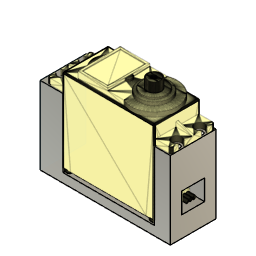
MG996R bracket(bairing) v1 (Autodesk Fusion 360 design; units mm, degrees)
Autodesk Fusion 360 part; units mm, degrees
other "基準メッシュ フィーチャ1"
other "修正1"
other "修正2"
sketch "スケッチ1" plane through (0, 0, 0) normal (0, 0, 1) x (1, 0, 0)
other "修正3"
sketch "スケッチ2" plane through (0, 0, 0) normal (0, 0, 1) x (1, 0, 0)
  line L0 (-20, 10) -> (20, 10)
  line L1 (20, 10) -> (20, -10)
  line L2 (20, -10) -> (-20, -10)
  line L3 (-20, -10) -> (-20, 10)
  line L4 (-20, 10) -> (20, -10) construction
  line L5 (20, 10) -> (-20, -10) construction
  line L6 (20, -10) -> (27, -10)
  line L7 (27, -10) -> (27, 10)
  line L8 (27, 10) -> (20, 10)
  line L9 (20, 10) -> (20, -10)
  line L10 (-20, -10) -> (-27, -10)
  line L11 (-27, -10) -> (-27, 10)
  line L12 (-27, 10) -> (-20, 10)
  line L13 (-20, 10) -> (-20, -10)
  dimension "d1" = 7
  dimension "d2" = 20
  dimension "d3" = 7
  dimension "d4" = 20
  constraint horizontal L0
  constraint perpendicular L0 L1
  constraint parallel L0 L2
  constraint parallel L1 L3
  constraint coincident L4 origin
  constraint coincident L5 origin
  constraint horizontal L6
  constraint vertical L7
  constraint horizontal L8
  constraint vertical L9
  constraint horizontal L10
  constraint vertical L11
  constraint horizontal L12
  constraint vertical L13
  measures "d1" distance of L1.end L6.end
  measures "d2" distance of L1.end L0.end
  measures "d3" distance of L2.end L10.end
  measures "d4" distance of L2.end L0.start
extrude "押し出し1" add sketch "スケッチ2" along normal blind 3
sketch "スケッチ3" plane through (0, 0, 3) normal (0, 0, 1) x (-1, 0, 0)
  line L0 (27, 10) -> (-27, 10)
  line L1 (-27, 10) -> (-27, -10)
  line L2 (-27, -10) -> (27, -10)
  line L3 (27, -10) -> (27, 10)
  line L4 (27, 10) -> (20, 10)
  line L5 (20, 10) -> (20, -10)
  line L6 (20, -10) -> (27, -10)
  line L7 (27, -10) -> (27, 10)
  line L8 (-27, 10) -> (-20, 10)
  line L9 (-20, 10) -> (-20, -10)
  line L10 (-20, -10) -> (-27, -10)
  line L11 (-27, -10) -> (-27, 10)
  constraint horizontal L4
  constraint vertical L5
  constraint horizontal L6
  constraint vertical L7
  constraint coincident L2 L5.end
  constraint coincident L0.start L3.end
  constraint horizontal L8
  constraint vertical L9
  constraint horizontal L10
  constraint vertical L11
  constraint coincident L0.end L1.start
extrude "押し出し2" add sketch "スケッチ3" along normal blind 5 contours L0 L2 L3 L4 L5 L6 L7 | L0 L1 L2 L8 L9 L10 L11
sketch "スケッチ4" plane through (0, 0, 8) normal (0, 0, 1) x (-1, 0, 0)
  line L0 (-27, -10) -> (-20, -10)
  line L1 (-20, -10) -> (-20, 10)
  line L2 (-20, 10) -> (-27, 10)
  line L3 (-27, 10) -> (-27, -10)
  line L4 (-20, 10) -> (-27, 10)
  line L5 (-27, 10) -> (-27, 5)
  line L6 (-27, 5) -> (-20, 5)
  line L7 (-20, 5) -> (-20, 10)
  line L8 (-27, -10) -> (-20, -10)
  line L9 (-20, -10) -> (-20, -5)
  line L10 (-20, -5) -> (-27, -5)
  line L11 (-27, -5) -> (-27, -10)
  dimension "d9" = 7
  dimension "d10" = 5
  constraint horizontal L4
  constraint vertical L5
  constraint horizontal L6
  constraint vertical L7
  constraint coincident L3 L5.end
  constraint coincident L1.end L2.start
  constraint horizontal L8
  constraint vertical L9
  constraint horizontal L10
  constraint vertical L11
  constraint coincident L0.start L3.end
  measures "d9" distance of L0.start L0.end
  measures "d10" distance of L0.start L10.end
extrude "押し出し3" add sketch "スケッチ4" along normal blind 9 contours L0 L1 L3 L8 L9 L10 L11 | L1 L2 L3 L4 L5 L6 L7
sketch "スケッチ5" plane through (0, 0, 17) normal (0, 0, 1) x (-1, 0, 0)
  line L0 (-27, -5) -> (-27, -10)
  line L1 (-27, -10) -> (-20, -10)
  line L2 (-20, -10) -> (-20, -5)
  line L3 (-20, -5) -> (-27, -5)
  line L4 (-20, 10) -> (-27, 10)
  line L5 (-27, 10) -> (-27, -10)
  line L6 (-27, -10) -> (-20, -10)
  line L7 (-20, -10) -> (-20, 10)
  constraint horizontal L4
  constraint vertical L5
  constraint horizontal L6
  constraint vertical L7
  constraint coincident L0.end L1.start
extrude "押し出し4" add sketch "スケッチ5" along normal blind 16
extrude "押し出し5" add 1 faces at (-22.3333, 3.3333, 8) along direction (0, 0, 1) blind 25
sketch "スケッチ6" plane through (0, 0, 33) normal (0, 0, 1) x (-1, 0, 0)
  line L0 (-20, -10) -> (-20, 10)
  line L1 (-20, 10) -> (-27, 10)
  line L2 (-27, 10) -> (-27, -10)
  line L3 (-27, -10) -> (-20, -10)
  circle A0 centre (-25, 5) radius 1.5
  circle A1 centre (-25, -5) radius 1.5
  circle A2 centre (24.95, 5.2) radius 1.5
  circle A3 centre (25, -4.8) radius 1.5
  dimension "d17" = 3
  dimension "d18" = 3
  dimension "d19" = 3
  dimension "d20" = 3
  measures "d17" diameter of A0
  measures "d18" diameter of A1
  measures "d19" diameter of A2
  measures "d20" diameter of A3
extrude "押し出し6" cut sketch "スケッチ6" against normal blind 5 contours A0 | A1 | A2 | A3
thread "ねじ1" "ISO Metric profile 3.0 M3x0.5 M3x0.5 6H" major diameter 3.086 minor diameter 2.529 pitch 0.5 angle 60 resizes the face on face at (-26.4981, 4.8748, 29.6667)
thread "ねじ2" "ISO Metric profile 3.0 M3x0.5 M3x0.5 6H" major diameter 3.086 minor diameter 2.529 pitch 0.5 angle 60 resizes the face on face at (-26.4481, -5.1252, 29.6667)
thread "ねじ3" "ISO Metric profile 3.0 M3x0.5 M3x0.5 6H" major diameter 3.086 minor diameter 2.529 pitch 0.5 angle 60 resizes the face on face at (23.5019, -4.9252, 29.6667) on face at (23.5019, 5.0748, 29.6667)
extrude "押し出し7" add 1 faces at (-9, -3.3333, 0) along direction (0, 0, -1) blind 1
sketch "スケッチ7" plane through (0, 0, 0) normal (0, 0, 1) x (1, 0, 0)
  line L0 (-20, -10) -> (10.1, -10)
  line L1 (10.1, -10) -> (10.1, 10)
  line L2 (10.1, 10) -> (-20, 10)
  line L3 (-20, 10) -> (-20, -10)
  circle A0 centre (10.1, 0) radius 7
  dimension "d31" = 30.1
  dimension "d32" = 14
  constraint horizontal L0
  constraint vertical L1
  constraint horizontal L2
  constraint vertical L3
  constraint midpoint L1 A0.centre
  measures "d31" distance of L0.start L0.end
  measures "d32" diameter of A0
move_body "移動1" bodies 1 to x (1, 0, 0) y (0, 1, 0) z (0, 0, 1) at (0, 0, 1)
other "修正4"
extrude "押し出し8" cut sketch "スケッチ7" along normal blind 4 contours L1 A0 | L1 A0
extrude "押し出し9" add 1 faces at (-27, -3.3333, 11.3333) along direction (-1, 0, 0) blind 3
sketch "スケッチ8" plane through (-30, 0, 0) normal (-1, 0, 0) x (0, -1, 0)
  line L0 (10, 0) -> (10, 34)
  line L1 (10, 34) -> (-10, 34)
  line L2 (-10, 34) -> (-10, 0)
  line L3 (-10, 0) -> (10, 0)
